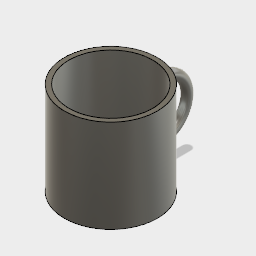
TEST4 (Autodesk Fusion 360 design; units mm, degrees)
Autodesk Fusion 360 part; units mm, degrees
cylinder "圆柱体基本要素1" add diameter 20 height 20 placed x (1, 0, 0) y (0, 0, -1) z (0, 1, 0) at (0, 0, 0) makes body 1
cylinder "圆柱体基本要素2" add diameter 18 height 20 placed x (0, 0, -1) y (0, 1, 0) z (1, 0, 0) at (0, 35, 60) separate body makes body 2
torus "圆环体基本要素1" add centre line diameter 12 section diameter 2 placed x (0, 0, -1) y (0, 1, 0) z (1, 0, 0) at (0, 33.1481, -24.3739) separate body makes body 3
move_body "MoveFace1" bodies 3 to x (1, 0, 0) y (0, 1, 0) z (0, 0, 1) at (0, -23, 14) on bodies 3
combine "合并1" operation add target body 3 tool bodies 1
move_body "对齐1" bodies 2 to x (0, 1, 0) y (0, 0, 1) z (1, 0, 0) at (-60, 0, -35)
extrude "拉伸1" cut 1 faces at (5.1676, 0, 0.3267) along direction (0, 1, 0) blind 2 on bodies 2 bodies 2
combine "合并2" operation cut target body 3 tool bodies 2
